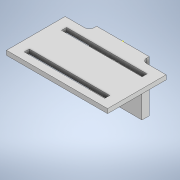
# Autodesk Inventor part: ServoESP32Base2
Saved by Autodesk Inventor 2020 (Build 240168000, 168)
## iProperties
Created: 2022-11-30
Part Number: ServoESP32Base2
Material: Generic
Document SubType Name: Modeling
Designer: agraa4529
Density: 1 g/cm^3
Appearance: Default
Author: agraa4529
## iProperties of the stored document _3DPrint.ipt
Created: 2022-12-02
Part Number: _3DPrint
Material: Generic
Document SubType Name: Modeling
Designer: agraa4529
Density: 1 g/cm^3
Appearance: Default
Author: agraa4529
Autodesk Inventor part; units mm, degrees
ref_plane "YZ Plane" through (0, 0, 0) normal (1, 0, 0) x (0, 1, 0)
ref_plane "XZ Plane" through (0, 0, 0) normal (0, 1, 0) x (-1, 0, 0)
ref_plane "XY Plane" through (0, 0, 0) normal (0, 0, 1) x (1, 0, 0)
sketch "Sketch1" plane through (0, 0, 0) normal (0, 0, 1) x (1, 0, 0)
  line L0 (-16, -16) -> (16, -16)
  line L1 (16, -16) -> (16, 16)
  line L2 (16, 16) -> (-16, 16)
  line L3 (-16, 16) -> (-16, -16)
  line L4 (-16, -16) -> (16, 16) construction
  line L5 (16, -16) -> (-16, 16) construction
  point P0 (0, 0)
  dimension "d1" = 32
  dimension "d2" = 32
  constraints: 12 end point, 2 midpoint, 2 parallel, 1 horizontal, 1 perpendicular
  measures "d1" distance of L2.end L1.end
  measures "d2" distance of L0.end L1.end
extrude "Extrusion1" add sketch "Sketch1" along normal blind 5
sketch "Sketch2" plane through (0, 0, 5) normal (0, 0, 1) x (1, 0, 0)
  line L0 (0, 0) -> (9.5, 0) construction
  circle A0 centre (9.5, 0) radius 1.5
  line L1 (0, 0) -> (0, 9.5) construction
  circle A1 centre (0, 9.5) radius 1.5
  line L2 (0, 0) -> (-9.5, 0) construction
  circle A2 centre (-9.5, 0) radius 1.5
  line L3 (0, 0) -> (0, -9.5) construction
  circle A3 centre (0, -9.5) radius 1.5
  dimension "d5" = 3
  dimension "d6" = 9.5
  dimension "d9" = 360
  constraints: 8 end point, 6 coincident, 4 centre point, 1 horizontal, 19 other
  measures "d5" diameter of A0
  measures "d6" distance of L0.start L0.end
extrude "Extrusion2" cut sketch "Sketch2" against normal blind 5
sketch "Sketch3" plane through (0, 0, 5) normal (0, 0, 1) x (1, 0, 0)
  circle A0 centre (0, 9.5) radius 1.5 projected
  circle A1 centre (0, 9.5) radius 3.1
  circle A2 centre (-9.5, 0) radius 3.1
  circle A3 centre (0, -9.5) radius 3.1
  circle A4 centre (9.5, 0) radius 3.1
  point P0 (0, 0)
  dimension "d13" = 6.2
  dimension "d16" = 360
  constraints: 4 centre point, 1 coincident, 9 other
  measures "d13" diameter of A1
extrude "Extrusion3" cut sketch "Sketch3" against normal blind 2.5
sketch "Sketch5" plane through (0, 0, 5) normal (0, 0, 1) x (1, 0, 0)
  circle A0 centre (0, 0) radius 3
  dimension "d25" = 6
  constraints: 1 centre point, 1 coincident
  measures "d25" diameter of A0
extrude "Extrusion5" cut sketch "Sketch5" against normal blind 10
sketch "Sketch8" plane through (0, 0, 0) normal (0, 0, -1) x (-1, 0, 0)
  line L0 (16, -16) -> (-16, -16) projected
  line L1 (-16, -16) -> (16, -16)
  line L2 (-16, 16) -> (16, 16) projected
  line L3 (-16, 16) -> (16, 16)
  line L4 (16, 16) -> (16, 19)
  line L5 (16, 19) -> (-16, 19)
  line L6 (-16, 19) -> (-16, 16)
  point P0 (0, 0)
  dimension "d32" = 32
  dimension "d33" = 3
  constraints: 10 end point, 2 horizontal, 2 parallel, 1 perpendicular
  measures "d32" distance of L4.end L5.end
  measures "d33" distance of L3.end L4.end
extrude "Extrusion6" add sketch "Sketch8" against normal blind 45
sketch "Sketch11" plane through (16, -16, 5) normal (1, 0, 0) x (0, 0, -1)
  line L0 (0, 0) -> (0, 32) projected
  line L1 (0, 32) -> (0, 0)
  line L2 (5, 0) -> (0, 0) projected
  line L3 (0, 0) -> (5, 0)
  line L4 (5, 0) -> (5, 35) projected
  line L5 (5, 0) -> (5, 35)
  line L6 (5, 35) -> (-40, 35) projected
  line L7 (5, 35) -> (-40, 35)
  line L8 (-40, 35) -> (-40, 32)
  line L9 (-40, 32) -> (0, 32)
  point P0 (5, 16)
  constraints: 12 end point, 5 perpendicular, 1 vertical
extrude "Extrusion9" add sketch "Sketch11" along normal blind 2
sketch "Sketch12" plane through (-16, -16, 0) normal (-1, 0, 0) x (0, 0, 1)
  line L0 (45, 32) -> (5, 32) projected
  line L1 (0, 0) -> (5, 0) projected
  line L2 (5, 32) -> (5, 0)
  line L3 (5, 0) -> (0, 0)
  line L4 (0, 35) -> (45, 35) projected
  line L5 (0, 0) -> (0, 35)
  line L6 (0, 35) -> (45, 35)
  line L7 (45, 35) -> (45, 32) projected
  line L8 (45, 35) -> (45, 32)
  line L9 (45, 32) -> (5, 32)
  point P0 (0, 16)
  constraints: 12 end point, 4 perpendicular, 2 collinear
extrude "Extrusion10" add sketch "Sketch12" along normal blind 2
sketch "Sketch13" plane through (-18, -16, 0) normal (-1, 0, 0) x (0, 0, 1)
  line L0 (45, 32) -> (5, 32) projected
  line L1 (5, 32) -> (45, 32)
  line L2 (45, 32) -> (45, 35)
  line L3 (45, 35) -> (5, 35)
  line L4 (5, 35) -> (5, 32)
  point P0 (0, 16)
  constraints: 8 end point, 2 parallel, 1 horizontal, 1 perpendicular
extrude "Extrusion11" add sketch "Sketch13" along normal blind 16.5
sketch "Sketch14" plane through (18, -16, 5) normal (1, 0, 0) x (0, 0, -1)
  line L0 (-40, 32) -> (0, 32) projected
  line L1 (-40, 35) -> (-40, 32) projected
  line L2 (0, 32) -> (-40, 32)
  line L3 (-40, 32) -> (-40, 35)
  line L4 (-40, 35) -> (0, 35)
  line L5 (0, 35) -> (0, 32)
  point P0 (5, 16)
  constraints: 8 end point, 2 parallel, 1 horizontal, 1 perpendicular
extrude "Extrusion12" add sketch "Sketch14" along normal blind 16.5
sketch "Sketch15" plane through (-18, 19, 0) normal (0, 1, 0) x (1, 0, 0)
  point P0 (18, 0)
sketch "Sketch16" plane through (-18, 19, 0) normal (0, 1, 0) x (1, 0, 0)
  line L0 (-16.5, -45) -> (52.5, -45) construction
  line L1 (36, -5) -> (52.5, -5) construction
  line L2 (-16.5, -45) -> (52.5, -45) construction
  line L3 (52.5, -45) -> (52.5, -5) construction
  line L4 (52.5, -5) -> (-16.5, -5) construction
  line L5 (-16.5, -5) -> (-16.5, -45) construction
  line L6 (-16.5, -4.9758) -> (-16.5, -45) construction
  line L7 (-16.5, -45) -> (52.5, -5) construction
  line L8 (0, -4.9758) -> (-16.5, -4.9758) construction
  line L9 (52.5, -5) -> (52.5, -45) construction
  line L10 (-16.5, -4.9758) -> (52.5, -45) construction
  line L11 (-9.5, -36.4633) -> (45.5, -36.4633) construction
  line L12 (45.5, -36.4633) -> (45.5, -14.4633) construction
  line L13 (45.5, -14.4633) -> (-9.5, -14.4633) construction
  line L14 (-9.5, -14.4633) -> (-9.5, -36.4633) construction
  line L15 (-9.5, -36.4633) -> (45.5, -14.4633) construction
  line L16 (45.5, -36.4633) -> (-9.5, -14.4633) construction
  line L17 (45.5, -14.4633) -> (-9.5, -14.4633)
  line L18 (-9.5, -14.4633) -> (-9.5, -10.9633)
  line L19 (-9.5, -10.9633) -> (45.5, -10.9633)
  line L20 (45.5, -10.9633) -> (45.5, -14.4633)
  line L21 (-9.5, -36.4633) -> (45.5, -36.4633)
  line L22 (45.5, -36.4633) -> (45.5, -39.9633)
  line L23 (45.5, -39.9633) -> (-9.5, -39.9633)
  line L24 (-9.5, -39.9633) -> (-9.5, -36.4633)
  point P0 (18, 0)
  point P1 (18, -25.4633)
  point P2 (0, -45)
  dimension "d57" = 55
  dimension "d58" = 22
  dimension "d59" = 3.5
  dimension "d60" = 3.5
  constraints: 40 end point, 8 parallel, 4 horizontal, 4 perpendicular, 2 midpoint, 1 point on line
  measures "d57" distance of L13.end L12.end
  measures "d58" distance of L11.end L12.end
  measures "d59" distance of L17.end L18.end
  measures "d60" distance of L21.end L22.end
extrude "Extrusion13" cut sketch "Sketch16" against normal blind 16.5
fillet "Fillet2" radius 3 1 edges at (0, 16, 5)
fillet "Fillet3" radius 3 4 edges at (18, 17.5, 5) (18, 16, 6.5) (-18, 16, 6.5) (-18, 17.5, 5)
body "Solid1"
